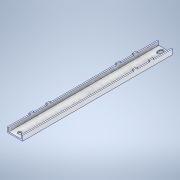
# Autodesk Inventor part: Barra fijación calefactor
Saved by Autodesk Inventor 2020 (Build 240168000, 168)
## iProperties
Created: 2020-06-08
Part Number: Barra fijación calefactor
Material: Aluminum 6061
Document SubType Name: Modeling
Designer: Bruno
Density: 2.7 g/cm^3
Appearance: Aluminum - Flat
Author: Bruno
Autodesk Inventor part; units mm, degrees
ref_plane "YZ Plane" through (0, 0, 0) normal (1, 0, 0) x (0, 1, 0)
ref_plane "XZ Plane" through (0, 0, 0) normal (0, 1, 0) x (-1, 0, 0)
ref_plane "XY Plane" through (0, 0, 0) normal (0, 0, 1) x (1, 0, 0)
sketch "Sketch1" plane through (0, 0, 0) normal (0, 1, 0) x (-1, 0, 0)
  line L0 (0, 0) -> (12, 0)
  line L1 (12, 0) -> (12, -119.5)
  line L2 (12, -119.5) -> (0, -119.5)
  line L3 (0, -119.5) -> (0, 0)
  circle A0 centre (6, -3.7) radius 1.4
  line L4 (6, -113.3) -> (6, -113.3)
  line L5 (4.6, -114.7) -> (4.6, -116.9)
  line L6 (6, -118.3) -> (6, -118.3)
  line L7 (7.4, -116.9) -> (7.4, -114.7)
  arc A1 (7.4, -114.7) -> (6, -113.3) centre (6, -114.7) ccw
  arc A2 (6, -118.3) -> (7.4, -116.9) centre (6, -116.9) ccw
  arc A3 (6, -113.3) -> (4.6, -114.7) centre (6, -114.7) ccw
  arc A4 (4.6, -116.9) -> (6, -118.3) centre (6, -116.9) ccw
  point P0 (4.6, -118.3)
  point P1 (4.6, -113.3)
  dimension "d0" = 12
  dimension "d1" = 119.5
  dimension "d2" = 2.8
  dimension "d3" = 5
  dimension "d4" = 1.4
  dimension "d5" = 2.8
  dimension "d6" = 3.7
  dimension "d7" = 6
  dimension "d8" = 1.2
  dimension "d9" = 6
  constraints: 16 end point, 8 point on circle, 8 tangent, 5 centre point, 4 parallel, 4 point on line, 3 equal radius, 2 horizontal, 2 perpendicular
  measures "d0" distance of L1.end L2.end
  measures "d1" distance of L0.end L1.end
  measures "d2" diameter of A0
  measures "d3" distance of point (4.6, -118.3) point (4.6, -113.3)
  measures "d4" radius of A1
  measures "d5" distance between parallel lines of L5 L7
  measures "d6" distance from line of L0 A0.centre
  measures "d7" distance from line of L3 A0.centre
  measures "d8" distance from line of L2 L6.end
  measures "d9" distance from line of L3 A1.centre
extrude "Extrusion1" add sketch "Sketch1" along normal blind 4
sketch "Sketch2" plane through (-12, 0, 0) normal (0, 0, 1) x (1, 0, 0)
  line L0 (12, 4) -> (0, 4) projected
  line L1 (1, 4) -> (11, 4)
  line L2 (11, 4) -> (11, 1)
  line L3 (11, 1) -> (1, 1)
  line L4 (1, 1) -> (1, 4)
  line L5 (0, 0) -> (0, 4) projected
  line L6 (12, 0) -> (12, 4) projected
  line L7 (0, 0) -> (12, 0) projected
  dimension "d12" = 1
  dimension "d13" = 1
  dimension "d14" = 1
  constraints: 8 end point, 2 parallel, 1 horizontal, 1 perpendicular, 1 point on line
  measures "d12" distance between parallel lines of L5 L4
  measures "d13" distance between parallel lines of L6 L2
  measures "d14" distance between parallel lines of L7 L3
extrude "Extrusion2" cut sketch "Sketch2" against normal through all contours L2 L3 L4 L0
sketch "Sketch3" plane through (0, 4, 0) normal (0, 1, 0) x (1, 0, 0)
  line L0 (-12, 119.5) -> (-12, 0) projected
  line L1 (-11, 0) -> (-11, 119.5) projected
  line L2 (-12, 17) -> (-11, 17)
  line L3 (-11, 17) -> (-11, 20)
  line L4 (-11, 20) -> (-12, 20)
  line L5 (-12, 20) -> (-12, 17)
  line L6 (-12, 30.5) -> (-11, 30.5)
  line L7 (-11, 30.5) -> (-11, 33.5)
  line L8 (-11, 33.5) -> (-12, 33.5)
  line L9 (-12, 33.5) -> (-12, 30.5)
  line L10 (-12, 86) -> (-11, 86)
  line L11 (-11, 86) -> (-11, 89)
  line L12 (-11, 89) -> (-12, 89)
  line L13 (-12, 89) -> (-12, 86)
  line L14 (-12, 99.5) -> (-11, 99.5)
  line L15 (-11, 99.5) -> (-11, 102.5)
  line L16 (-11, 102.5) -> (-12, 102.5)
  line L17 (-12, 102.5) -> (-12, 99.5)
  line L18 (-1, 0) -> (-1, 119.5) projected
  line L19 (0, 0) -> (0, 119.5) projected
  line L20 (0, 99.5) -> (0, 102.5)
  line L21 (-1, 102.5) -> (-1, 99.5)
  line L22 (-1, 88.5) -> (0, 88.5)
  line L23 (0, 88.5) -> (0, 91.5)
  line L24 (0, 91.5) -> (-1, 91.5)
  line L25 (-1, 91.5) -> (-1, 88.5)
  line L26 (-12, 0) -> (-11, 0) projected
  line L27 (-11, 119.5) -> (-12, 119.5) projected
  line L28 (0, 119.5) -> (-1, 119.5) projected
  line L29 (-1, 104.5) -> (0, 104.5)
  line L30 (0, 104.5) -> (0, 101.5)
  line L31 (0, 101.5) -> (-1, 101.5)
  line L32 (-1, 101.5) -> (-1, 104.5)
  point P0 (0, 88.5)
  dimension "d17" = 3
  dimension "d18" = 17
  dimension "d19" = 3
  dimension "d20" = 3
  dimension "d21" = 3
  dimension "d22" = 3
  dimension "d24" = 10.5
  dimension "d25" = 17
  dimension "d26" = 10.5
  dimension "d28" = 1
  dimension "d29" = 3
  dimension "d30" = 15
  dimension "d31" = 10
  constraints: 52 end point, 14 point on line, 13 parallel, 6 horizontal, 6 perpendicular
  measures "d17" distance of L4.end L2.start
  measures "d18" distance between parallel lines of L26 L2
  measures "d19" distance between parallel lines of L8 L6
  measures "d20" distance between parallel lines of L12 L10
  measures "d21" distance between parallel lines of L16 L14
  measures "d22" distance between parallel lines of L24 L22
  measures "d24" distance between parallel lines of L6 L4
  measures "d25" distance between parallel lines of L27 L16
  measures "d26" distance between parallel lines of L14 L12
  measures "d28" distance of L30.end L31.end
  measures "d29" distance of L29.end L30.end
  measures "d30" distance between parallel lines of L28 L29
  measures "d31" distance between parallel lines of L24 L31
extrude "Extrusion3" add sketch "Sketch3" along normal blind 1 contours L16 L1 L14 L0 | L12 L1 L10 L0 | L8 L1 L6 L0 | L4 L1 L2 L0 | L18 L24 L19 L22 | L18 L29 L19 L31
sketch "Sketch4" plane through (0, 4, 0) normal (0, 1, 0) x (1, 0, 0)
  line L0 (0, 119.5) -> (-12, 119.5) projected
  line L1 (-6, 119.5) -> (-6, 59.75) construction
  line L2 (-1, 0) -> (-11, 0) projected
  circle A0 centre (-6, 3.7) radius 1.4 projected
  circle A1 centre (-6, 59.75) radius 56.05 construction
  point P0 (0, 0)
  dimension "d34" = 59.75
  constraints: 2 end point, 1 coincident, 1 midpoint, 1 perpendicular, 1 vertical alignment, 2 other
  measures "d34" distance of L1.start L1.end
equation "\"d19\" = d17"
equation "\"d20\" = d17"
equation "\"d21\" = d17"
equation "\"d22\" = d17"
body "Solid1"
